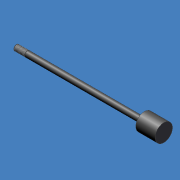
# Autodesk Inventor part: 043.5-DQ0_rod
Saved by Autodesk Inventor 2012 (Build 160160000, 160)
## iProperties
Category: PARTsolutions
Created: 2013-01-20
Part Number: 043.5-DQ0_rod
Catalog Web Link: www.cadenas.de
Description: Standard Air Cylinder_rod - Original Line - Standard Air Cylinders
Document SubType Name: Modeling
Designer: PARTsolutions
Material: Default
Density: 1 g/cm^3
Mass: 10.7362 g
Surface Area: 47.1599 cm^2
Volume: 10.7362 cm^3
NB: 043.5-DQ0_rod
NN: Standard Air Cylinder_rod
NT: Original Line - Standard Air Cylinders
NBSYN: $PN.$COLOR1._rod
LINA: 043.5-DQ0_rod
PN: 043.5-DQ
DASH: -
BORE: 0.75000000
BOREPN: 04
STROKE: 3.500
STROKEALG: [0.001:50/0.001]
STROKE1: 3.500
ACTING: D
ACTINGALG: '' , 'Single Acting' , 'R' , 'Reverse Single Acting' , 'D' , 'Double Acting'
ACTINGPN: D
MNTALG: '' , 'Front Nose Mounting' , 'P' , 'Rear Pivot Mounting' , 'XP' , 'Double End or Pivot Mounting' , 'X' , 'Double End Mounting' , 'BF' , 'Front Block Mounting' , 'BR' , 'Rear Block Mounting for Vertical Positioning' , 'BFT' , 'Front Block Trunnion Mounting' , 'BRT' , 'Rear Block Trunnion Mounting'
DERALG: '' , 'N/A'
NRALG: '' , 'N/A'
BMALG: '' , 'N/A'
COALG: '' , 'N/A'
MALG: '', 'Without Magnet', 'M', 'With Magnet'
EEL: 0
EEMAX: 8
EEALG: '', 'Without Extra Extension', 'EE', 'With Extra Extension'
EELALG: 0
EEPN1: 0.000
KALG: '' , 'N/A'
Q: Q
QALG: '' , 'Without Side Ported Rear Head' , 'Q' , 'With Side Ported Rear Head'
QPN: Q
YALG: '' , 'N/A'
FALG: '', 'Standard', 'F', 'Molycoated Body'
TALG: '' , 'Standard' , 'N' , 'Low Temperature' , 'V' , 'High Temperature'
BALG: '', 'Without Bumper' , 'B' , 'With Bumper'
HALG: '', 'N/A'
SERALG: '' , 'Without Spring Extend/Return' , 'JS' , 'With Spring Return' , 'JR' , 'With Spring Extend'
SR: C
SRALG: 'C' , 'Carbon Steel Rod' , 'SR' , '303 Stainless Steel Rod' , '' , '303 Stainless Steel Rod1'
SRCON: 1
WALG: '' , 'Without Wiper' , 'W' , 'With Wiper'
EALG: '' , 'Without Special Lube and Seals' , 'E' , 'With Special Lube and Seals'
HLALG: '' , 'Wihout Low Pressure Hydraulic' , 'HL' , 'With Low Pressure Hydraulic'
STALG: '' , 'Without Switch Track' , 'T' , 'With Switch Track'
STPALG: '' , 'N/A'
PRCALG: '' , 'Without Piston Rod Clevis' , 'D-166-1' , 'With Piston Rod Clevis'
PBALG: '' , 'Without Pivot Bracket' , 'D-167' , 'With Pivot Bracket'
TLEN: 4.7565
TEXT: 0.333
SPACE: 0.190
FRAC: 16.4700
RGDACCON: R
RHCONON: 1
FNUTCON: 1
RNUTCON: 0
FNUTPN: D-9
FNUTTRANS: 0.0000
RNUTTRANS: 0.0000
VHOLECON: 0
A1: 1.5940
A1N: 0.8750
A1P: 1.5940
A1B: 1.5940
A4: 0.2525
A4N: 0.3130
A4P: 0.2525
A5: 0.0300
A1H: 0.531
A1NH: 0.5310
A1PH: 1.5940
A1BH: 1.0940
A1SH: 1.2190
A2H: 0.2190
A2NH: 0.2190
LENGTH: 2.9700
LENGTH1: 2.9700
LENGTH2: 3.0300
MUL: 3.5000
MUL11: 3.5000
MUL22: 9.4150
MUL33: 5.9150
MUL2: 3.5000
MUL211: 3.5000
MUL222: 2.6900
MUL233: 1.6900
SSS: 7.0000
RGLEN: 1.3715
RHLEN: 0.3420
SSS1: 4.0000
A13: 1.3120
THDLEN1: 0.5000
THD1: 0.2500
TAB: UNF
THDLEN: 0.5000
THD: 0.2500
OD: 0.7615
RODL: 6.4390
PL: 0.8450
RODDIA: 0.2500
HEX: 0.2500
RODTRANS: 0.0000
G1: 0.1250
ON: 0
G5: 0.6250
DERLEN: 5.5940
THOLE: 0.0000
WF: 0.2200
BADD: 0.0000
MADD: 0.0000
NVADD: 0.000
JRADD: 0.00000
COLOR: 0.00,0.00,0.00,0.00
GROOVE: 1
HOL: 0
D7: 0.2520
H1: 1.1175
D1: 0.8625
D1RH: 0.8050
D1P: 0.8325
D1B: 0.8625
D1N: 0.8050
D1NRH: 0.8050
D1BRH: 0.8325
D1PRH: 0.8625
BOZO: 1
HADD: 0.000
COLOR1: 0
DEFL: 0.0000
HEXL: 0.0000
SSADD: 0.0000
WFL: 0.0000
MOVE: 0.0000
KT: DUMMY
SUPPLIER: Bimba
ARTICLENO: 043.5-DQ0_rod
BOMINFO: 043.5-DQ0_rod
CREATOR: CADENAS GmbH
PSOL_IDENT_0: {\\10.0.0.242\data_v9\23d-libs\bimba\bimba\bimba_imperial\bimba_full_line\original_line_cylinders\st
PSOL_IDENT_1: andard_air_cylinders\rod.prj},280 {VTYP=3D},{NB=043.5-DQ0_rod},{LINA=043.5-DQ0_rod},{NN=Standard Air
PSOL_IDENT_2: Cylinder_rod},{DATE=11.09.2012 07:37:40},{GEOMDATE=06.09.2012 09:06:00},{VERSION=},{LINEID=50},{LIN
PSOL_IDENT_3: ESUBID=-1},{WBVAR=STROKE,ACTING,MNT,DER,NR,BM,CO,M,EE,EEL,K,Q,Y,F,G,T,B,H,SER,SR,NT,W,E,HL,ST,STP,PR
PSOL_IDENT_4: C,PB,COLOR1}  {NB=043.5-DQ0_rod},{LINA=043.5-DQ0_rod},{KT=DUMMY},{PN=043.5-DQ},{DASH=-},{BORE=0.7500
PSOL_IDENT_5: 0000},{BOREPN=04},{STROKE=3.500},{STROKEALG=[0.001:50/0.001]},{STROKE1=3.500},{ACTING=D},{ACTINGALG=
PSOL_IDENT_6: '' , 'Single Acting' , 'R' , 'Reverse Single Acting' , 'D' , 'Double Acting' },{ACTINGPN=D},{MNT=},
PSOL_IDENT_7: {MNTALG= '' , 'Front Nose Mounting' , 'P' , 'Rear Pivot Mounting' , 'XP' , 'Double End or Pivot Moun
PSOL_IDENT_8: ting' , 'X' , 'Double End Mounting' , 'BF' , 'Front Block Mounting' , 'BR' , 'Rear Block Mounting fo
PSOL_IDENT_9: r Vertical Positioning' , 'BFT' , 'Front Block Trunnion Mounting' , 'BRT' , 'Rear Block Trunnion Mou
PSOL_IDENT_10: nting' },{TYPE=},{MNTPN=},{DER=},{DERALG= '' , 'N/A' },{NR=},{NRALG= '' , 'N/A' },{NRPN=},{BM=},{BMA
PSOL_IDENT_11: LG= '' , 'N/A' },{BMPN=},{CO=},{COALG= '' , 'N/A' },{M=},{MALG= '', 'Without Magnet', 'M', 'With Mag
PSOL_IDENT_12: net' },{EE=},{EEL=0},{EEMAX=8},{EEALG= '', 'Without Extra Extension', 'EE', 'With Extra Extension' }
PSOL_IDENT_13: ,{EELALG=0},{EEPN=},{EEPN1=0.000},{K=},{KALG= '' , 'N/A' },{KPN=},{Q=Q},{QALG= '' , 'Without Side Po
PSOL_IDENT_14: rted Rear Head' , 'Q' , 'With Side Ported Rear Head' },{QPN=Q},{Y=},{YALG= '' , 'N/A' },{YPN=},{F=},
PSOL_IDENT_15: {FALG= '', 'Standard', 'F', 'Molycoated Body' },{FPN=},{G=},{GPN=},{T=},{TALG= '' , 'Standard' , 'N'
PSOL_IDENT_16: , 'Low Temperature' , 'V' , 'High Temperature' },{NPN=},{VPN=},{B=},{BALG= '', 'Without Bumper' , '
PSOL_IDENT_17: B' , 'With Bumper' },{BPN=},{H=},{HALG= '', 'N/A' },{HPN=},{SER=},{SERALG= '' , 'Without Spring Exte
PSOL_IDENT_18: nd/Return' , 'JS' , 'With Spring Return' , 'JR' , 'With Spring Extend' },{SR=C},{SRALG= 'C' , 'Carbo
PSOL_IDENT_19: n Steel Rod' , 'SR' , '303 Stainless Steel Rod' , '' , '303 Stainless Steel Rod1' },{SRPN=},{SRCON=1
PSOL_IDENT_20: },{NT=},{NTPN=},{W=},{WALG= '' , 'Without Wiper' , 'W' , 'With Wiper' },{WPN=},{E=},{EALG= '' , 'Wit
PSOL_IDENT_21: hout Special Lube and Seals' , 'E' , 'With Special Lube and Seals' },{EPN=},{HL=},{HLALG= '' , 'Wiho
PSOL_IDENT_22: ut Low Pressure Hydraulic' , 'HL' , 'With Low Pressure Hydraulic' },{ST=},{STALG= '' , 'Without Swit
PSOL_IDENT_23: ch Track' , 'T' , 'With Switch Track' },{STP=},{STPALG= '' , 'N/A' },{STPN=},{PRC=},{PRCALG= '' , 'W
PSOL_IDENT_24: ithout Piston Rod Clevis' , 'D-166-1' , 'With Piston Rod Clevis' },{PRCPN=},{PB=},{PBALG= '' , 'With
PSOL_IDENT_25: out Pivot Bracket' , 'D-167' , 'With Pivot Bracket' },{PBPN=},{TLEN=4.7565},{TEXT=0.333333},{SPACE=0
PSOL_IDENT_26: .190476},{FRAC=16.4700},{RGCON=},{RGDACCON=R},{RHCON=},{RHCONON=1},{RHACCON=},{FNUTCON=1},{RNUTCON=0
PSOL_IDENT_27: },{FNUTPN=D-9},{RNUTPN=},{FNUTTRANS=0.0000},{RNUTTRANS=0.0000},{VHOLECON=0},{A1=1.5940},{A1N=0.8750}
PSOL_IDENT_28: ,{A1P=1.5940},{A1B=1.5940},{A4=0.2525},{A4N=0.3130},{A4P=0.2525},{A5=0.0300},{A1H=0.531},{A1NH=0.531
PSOL_IDENT_29: 0},{A1PH=1.5940},{A1BH=1.0940},{A1SH=1.2190},{A2H=0.2190},{A2NH=0.2190},{LENGTH=2.9700},{LENGTH1=2.9
PSOL_IDENT_30: 700},{LENGTH2=3.0300},{MUL=3.5000},{MUL11=3.5000},{MUL22=9.4150},{MUL33=5.9150},{MUL2=3.5000},{MUL21
PSOL_IDENT_31: 1=3.5000},{MUL222=2.6900},{MUL233=1.6900},{SSS=7.0000},{RGLEN=1.3715},{RHLEN=0.3420},{SSS1=4.0000},{
PSOL_IDENT_32: A13=1.3120},{THDLEN1=0.5000},{THD1=0.2500},{TAB=UNF},{THDLEN=0.5000},{THD=0.2500},{OD=0.7615},{RODL=
PSOL_IDENT_33: 6.4390},{PL=0.8450},{RODDIA=0.2500},{HEX=0.2500},{RODTRANS=0.0000},{G1=0.1250},{ON=0},{G5=0.6250},{D
PSOL_IDENT_34: ERLEN=5.5940},{THOLE=0.0000},{WF=0.2200},{BADD=0.0000},{MADD=0.0000},{NVADD=0.000},{JRADD=0.00000},{
PSOL_IDENT_35: COLOR=0.00,0.00,0.00,0.00},{GROOVE=1},{HOL=0},{D7=0.2520},{H1=1.1175},{D1=0.8625},{D1RH=0.8050},{D1P
PSOL_IDENT_36: =0.8325},{D1B=0.8625},{D1N=0.8050},{D1NRH=0.8050},{D1BRH=0.8325},{D1PRH=0.8625},{BOZO=1},{HADD=0.000
PSOL_IDENT_37: },{COLOR1=0},{DEFL=0.0000},{HEXL=0.0000},{SSADD=0.0000},{WFL=0.0000},{MOVE=0.0000}
Title: 043.5-DQ0_rod
Author: Cadenas PARTsolutions
Comments: Original Line - Standard Air Cylinders
Autodesk Inventor part; units mm, degrees
sketch "Sketch_1" plane through (0, 0, 0) normal (0, 0, 1) x (1, 0, 0)
  line L0 (150.8506, 0) -> (0, 0)
  line L1 (0, 0) -> (0, 3.175)
  line L2 (0, 3.175) -> (129.3876, 3.175)
  line L3 (129.3876, 3.175) -> (129.3876, 9.6203)
  line L4 (129.3876, 9.6203) -> (150.8506, 9.6203)
  line L5 (150.8506, 9.6203) -> (150.8506, 0)
  line L6 (150.8506, 0) -> (0, 0)
  constraints: 14 end point
revolve "Revolution1" add sketch "Sketch_1" angle 360 about axis through (150.8506, 0, 0) along (1, 0, 0)
sketch "Sketch_3" plane through (0, 0, 0) normal (0, 0, 1) x (1, 0, 0)
  line L0 (0, 0) -> (-12.7, 0)
  line L1 (-12.7, 0) -> (-12.7, 2.634)
  line L2 (-12.7, 2.634) -> (-12.159, 3.175)
  line L3 (-12.159, 3.175) -> (0, 3.175)
  line L4 (0, 3.175) -> (0, 0)
  line L5 (0, 0) -> (-12.7, 0)
  constraints: 12 end point
revolve "Revolution2" add sketch "Sketch_3" angle 360 about axis through (0, 0, 0) along (1, 0, 0)
thread "Thread1" size "1/4-28 UNF" class "3A" standard "ANSI Unified Screw Threads" length 12.7 offset 129.3876
sketch "Sketch_30" plane through (0, 0, 0) normal (0, 0, 1) x (1, 0, 0)
  line L0 (0, 0) -> (-0.254, 0)
  line L1 (-0.254, 3.429) -> (-0.254, 2.921)
  line L2 (-0.254, 2.921) -> (0, 2.921)
  line L3 (0, 2.921) -> (0, 3.429)
  line L4 (0, 3.429) -> (-0.254, 3.429)
  constraints: 10 end point
revolve "Revolution3" cut sketch "Sketch_30" angle 360 about axis through (0, 0, 0) along (1, 0, 0)
ref_plane "rod_cp_XY" through (0, 0, 0) normal (1, 0, 0) x (0, 0, -1)
ref_plane "rod_cp_YZ" through (0, 0, 0) normal (0, 0, -1) x (0, 1, 0)
ref_plane "rod_cp_ZX" through (0, 0, 0) normal (0, 1, 0) x (1, 0, 0)
ref_plane "to_rod_clevis_XY" through (-12.7, 0, 0) normal (1, 0, 0) x (0, 0, -1)
ref_plane "to_rod_clevis_YZ" through (-12.7, 0, 0) normal (0, 0, -1) x (0, 1, 0)
ref_plane "to_rod_clevis_ZX" through (-12.7, 0, 0) normal (0, 1, 0) x (1, 0, 0)
ref_plane "rl2_XY" through (0, 0, 0) normal (1, 0, 0) x (0, 0, -1)
ref_plane "rl2_YZ" through (0, 0, 0) normal (0, 0, -1) x (0, 1, 0)
ref_plane "rl2_ZX" through (0, 0, 0) normal (0, 1, 0) x (1, 0, 0)
ref_plane "rl1_XY" through (-12.7, 0, 0) normal (1, 0, 0) x (0, 0, -1)
ref_plane "rl1_YZ" through (-12.7, 0, 0) normal (0, 0, -1) x (0, 1, 0)
ref_plane "rl1_ZX" through (-12.7, 0, 0) normal (0, 1, 0) x (1, 0, 0)
ref_plane "thd1_XY" through (-12.7, 3.175, 0) normal (1, 0, 0) x (0, 0, -1)
ref_plane "thd1_YZ" through (-12.7, 3.175, 0) normal (0, 0, -1) x (0, 1, 0)
ref_plane "thd1_ZX" through (-12.7, 3.175, 0) normal (0, 1, 0) x (1, 0, 0)
ref_plane "thd2_XY" through (-12.7, -3.175, 0) normal (1, 0, 0) x (0, 0, -1)
ref_plane "thd2_YZ" through (-12.7, -3.175, 0) normal (0, 0, -1) x (0, 1, 0)
ref_plane "thd2_ZX" through (-12.7, -3.175, 0) normal (0, 1, 0) x (1, 0, 0)
ref_plane "dia1_XY" through (0, 3.175, 0) normal (1, 0, 0) x (0, 0, -1)
ref_plane "dia1_YZ" through (0, 3.175, 0) normal (0, 0, -1) x (0, 1, 0)
ref_plane "dia1_ZX" through (0, 3.175, 0) normal (0, 1, 0) x (1, 0, 0)
ref_plane "dia2_XY" through (0, -3.175, 0) normal (1, 0, 0) x (0, 0, -1)
ref_plane "dia2_YZ" through (0, -3.175, 0) normal (0, 0, -1) x (0, 1, 0)
ref_plane "dia2_ZX" through (0, -3.175, 0) normal (0, 1, 0) x (1, 0, 0)
ref_plane "dia1r_XY" through (0, 0, 10.2235) normal (1, 0, 0) x (0, 0, -1)
ref_plane "dia1r_YZ" through (0, 0, 10.2235) normal (0, 0, -1) x (0, 1, 0)
ref_plane "dia1r_ZX" through (0, 0, 10.2235) normal (0, 1, 0) x (1, 0, 0)
ref_plane "dia2r_XY" through (0, 0, -10.2235) normal (1, 0, 0) x (0, 0, -1)
ref_plane "dia2r_YZ" through (0, 0, -10.2235) normal (0, 0, -1) x (0, 1, 0)
ref_plane "dia2r_ZX" through (0, 0, -10.2235) normal (0, 1, 0) x (1, 0, 0)
ref_plane "dia12_XY" through (0, 0, 10.9537) normal (1, 0, 0) x (0, 0, -1)
ref_plane "dia12_YZ" through (0, 0, 10.9537) normal (0, 0, -1) x (0, 1, 0)
ref_plane "dia12_ZX" through (0, 0, 10.9537) normal (0, 1, 0) x (1, 0, 0)
ref_plane "dia22_XY" through (0, 0, -10.9537) normal (1, 0, 0) x (0, 0, -1)
ref_plane "dia22_YZ" through (0, 0, -10.9537) normal (0, 0, -1) x (0, 1, 0)
ref_plane "dia22_ZX" through (0, 0, -10.9537) normal (0, 1, 0) x (1, 0, 0)
body "Solid1"
